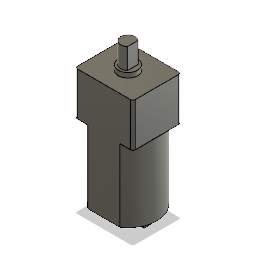
Pulley (Autodesk Fusion 360 archive; units mm, degrees)
design "VE508 Small Gear Motor"
Autodesk Fusion 360 part; units mm, degrees
sketch "Sketch1" plane through (0, 0, 0) normal (0, 1, 0) x (1, 0, 0) in component "Motor"
  line L0 (6, 5) -> (-6, 5)
  line L1 (-6, 5) -> (-6, -5)
  line L2 (-6, -5) -> (6, -5)
  line L3 (6, -5) -> (6, 5)
  line L4 (6, 5) -> (-6, -5) construction
  line L5 (-6, 5) -> (6, -5) construction
  dimension "d1" = 10
  dimension "d2" = 12
  constraint perpendicular L0 L1
  constraint parallel L0 L2
  constraint parallel L1 L3
  constraint horizontal L0
  constraint coincident L4 origin
  constraint coincident L5 origin
  measures "d1" distance of L0.end L1.end
  measures "d2" distance of L0.start L0.end
extrude "Extrude1" add sketch "Sketch1" against normal blind 9 makes body 1 in component "Motor"
sketch "Sketch2" plane through (0, -9, 0) normal (0, -1, 0) x (1, 0, 0) in component "Motor"
  line L0 (6, -5) -> (6, 5)
  line L1 (6, 5) -> (-6, 5)
  line L2 (-6, 5) -> (-6, -5)
  line L3 (-6, -5) -> (6, -5)
  circle A0 centre (0, 0) radius 6
  constraint coincident A0.centre origin
  constraint tangent L0 A0
extrude "Extrude2" add sketch "Sketch2" along normal blind 15 contours L1 L3 A0 bodies 1 in component "Motor"
sketch "Sketch3" plane through (0, -24, 0) normal (0, -1, 0) x (1, 0, 0) in component "Motor"
  arc A0 (3.3166, -5) -> (3.3166, 5) centre (0, 0) ccw
  line L0 (3.3166, 5) -> (-3.3166, 5)
  arc A1 (-3.3166, 5) -> (-3.3166, -5) centre (0, 0) ccw
  line L1 (-3.3166, -5) -> (3.3166, -5)
  circle A2 centre (0, 0) radius 2.5
  line L2 (-4, 0) -> (4, 0) construction
  line L3 (0, 5) -> (0, -5) construction
  line L4 (-4, 0.75) -> (-3.65, 0.75)
  line L5 (-3.65, 0.75) -> (-3.65, -0.75)
  line L6 (-3.65, -0.75) -> (-4, -0.75)
  line L7 (-4, -0.75) -> (-4, 0.75)
  line L8 (3.65, -0.75) -> (4, -0.75)
  line L9 (4, -0.75) -> (4, 0.75)
  line L10 (3.65, 0.75) -> (3.65, -0.75)
  line L11 (4, 0.75) -> (3.65, 0.75)
  dimension "d7" = 5
  dimension "d10" = 8
  dimension "d11" = 0.35
  dimension "d12" = 1.5
  constraint concentric A0 A2
  constraint horizontal L2
  constraint coincident A0.centre L2
  constraint midpoint L0 L3.start
  constraint midpoint L1 L3.end
  constraint symmetric L2.start L2.end L3
  constraint horizontal L4
  constraint vertical L5
  constraint horizontal L6
  constraint vertical L7
  constraint coincident L2.start L7
  constraint symmetric L2 L4 L6
  constraint symmetric L3 L4.start L9.end
  constraint symmetric L3 L4.end L10.start
  constraint symmetric L3 L5.end L8.start
  constraint symmetric L3 L6.end L8.end
  measures "d7" diameter of A2
  measures "d10" distance of L2.start L2.end
  measures "d11" distance of L5.end L6.end
  measures "d12" distance of L4.start L6.end
extrude "Extrude4" add sketch "Sketch3" along normal blind 2 contours L4 L5 L6 L7 | L8 L9 L10 L11 bodies 1 in component "Motor"
extrude "Extrude3" add sketch "Sketch3" along normal blind 1 contours A2 bodies 1 in component "Motor"
fillet "Fillet1" radius 0.5 4 edges at (6, -4.5, -5) (-6, -4.5, -5) (-6, -4.5, 5) (6, -4.5, 5) on bodies 1 in component "Motor"
sketch "Sketch4" plane through (0, 0, 0) normal (0, 1, 0) x (-1, 0, 0) in component "Motor"
  arc A0 (-5.5, 5) -> (-6, 4.5) centre (-5.5, 4.5) ccw
  line L0 (-6, 4.5) -> (-6, -4.5)
  arc A1 (-6, -4.5) -> (-5.5, -5) centre (-5.5, -4.5) ccw
  line L1 (-5.5, -5) -> (5.5, -5)
  arc A2 (5.5, -5) -> (6, -4.5) centre (5.5, -4.5) ccw
  line L2 (6, -4.5) -> (6, 4.5)
  arc A3 (6, 4.5) -> (5.5, 5) centre (5.5, 4.5) ccw
  line L3 (5.5, 5) -> (-5.5, 5)
  circle A4 centre (0, 0) radius 2
  dimension "d16" = 4
  constraint coincident A4.centre origin
  measures "d16" diameter of A4
extrude "Extrude5" add sketch "Sketch4" along normal blind 1 contours A4 bodies 1 in component "Motor"
sketch "Sketch5" plane through (0, 1, 0) normal (0, 1, 0) x (-1, 0, 0) in component "Motor"
  circle A0 centre (0, 0) radius 2
  circle A1 centre (0, 0) radius 1.5
  line L0 (-1, -1.118) -> (-1, 1.118)
  line L1 (3.3166, -5) -> (-3.3166, -5) construction
  line L2 (5.5, 5) -> (-5.5, 5) construction
  line L3 (1.5, -5) -> (1.5, 5) construction
  dimension "d19" = 3
  dimension "d20" = 2.5
  constraint concentric A0 A1
  constraint coincident A1 L0.start
  constraint coincident A1 L0.end
  constraint coincident L1 L3.start
  constraint coincident L2 L3.end
  constraint tangent A1 L3
  constraint perpendicular L2 L3
  measures "d19" diameter of A1
  measures "d20" distance of L0 L3
extrude "Extrude6" add sketch "Sketch5" along normal blind 4.3 separate body contours A1 L0 picked at (-0.4625, 0.4564) makes body 2 in component "Motor"
copy_body "CutPasteBodies1" bodies 2 removing the originals makes body 3 in component "Rotor"
component "Motor" placed x (1, 0, 0) y (0, 1, 0) z (0, 0, 1) at (0, 0, 0)
component "Rotor" placed x (1, 0, 0) y (0, 1, 0) z (0, 0, 1) at (0, 0, 0)
